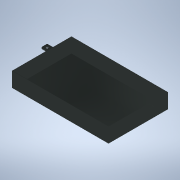
# Autodesk Inventor part: Soporte_Batería
Saved by Autodesk Inventor 2022.1 (Build 261234000, 234)
## iProperties
Part Number: Soporte_Batería
Material: Genérico
Document SubType Name: Modelado
Designer: seb_0
Appearance: Gris plomo - Pulido
Author: seb_0
Autodesk Inventor part; units mm, degrees
ref_plane "Plano YZ" through (0, 0, 0) normal (1, 0, 0) x (0, 1, 0)
ref_plane "Plano XZ" through (0, 0, 0) normal (0, 1, 0) x (-1, 0, 0)
ref_plane "Plano XY" through (0, 0, 0) normal (0, 0, 1) x (1, 0, 0)
sketch "Boceto1" plane through (0, 0, 0) normal (0, 1, 0) x (-1, 0, 0)
  line L0 (0, 0) -> (330.2, 0)
  line L1 (330.2, 0) -> (330.2, -200.66)
  line L2 (330.2, -200.66) -> (0, -200.66)
  line L3 (0, -200.66) -> (0, 0)
  line L4 (-1, -201.66) -> (331.2, -201.66)
  line L5 (331.2, -201.66) -> (331.2, 1)
  line L6 (331.2, 1) -> (-1, 1)
  line L7 (-1, 1) -> (-1, -201.66)
  dimension "d0" = 200.66
  dimension "d1" = 330.2
  dimension "d2" = 1
  constraints: 16 end point, 4 parallel, 2 perpendicular, 1 horizontal, 3 other
  measures "d0" distance of L2.end L0.start
  measures "d1" distance of L1.end L2.end
  measures "d2" distance between parallel lines of L2 L4
extrude "Extrusión1" add sketch "Boceto1" along normal blind 50
sketch "Boceto2" plane through (0, 0, 0) normal (0, -1, 0) x (1, 0, 0)
  line L0 (-331.2, 1) -> (1, 1) projected
  line L1 (1, 1) -> (1, -201.66) projected
  line L2 (-331.2, -201.66) -> (-331.2, 1) projected
  line L3 (1, -201.66) -> (-331.2, -201.66) projected
  point P0 (0, 0)
extrude "Extrusión2" add sketch "Boceto2" along normal blind 1
sketch "Boceto3" plane through (0, 50, 0) normal (0, 1, 0) x (1, 0, 0)
  line L0 (1, -1) -> (1, 201.66) projected
  line L1 (1, 140) -> (21, 140)
  line L2 (21, 140) -> (21, 120)
  line L3 (21, 120) -> (1, 120)
  line L4 (1, 120) -> (1, 140)
  line L5 (-331.2, -1) -> (1, -1) projected
  line L6 (-331.2, 201.66) -> (-331.2, -1) projected
  line L7 (-331.2, 140) -> (-351.2, 140)
  line L8 (-351.2, 140) -> (-351.2, 120)
  line L9 (-351.2, 120) -> (-331.2, 120)
  line L10 (-331.2, 120) -> (-331.2, 140)
  circle A0 centre (11, 130) radius 5
  line L11 (1, 140) -> (21, 120)
  line L12 (21, 140) -> (1, 120)
  line L13 (-351.2, 140) -> (-331.2, 120)
  line L14 (-331.2, 140) -> (-351.2, 120)
  circle A1 centre (-341.2, 130) radius 5
  point P0 (0, 0)
  point P1 (1, 120)
  dimension "d7" = 20
  dimension "d8" = 20
  dimension "d9" = 121
  dimension "d10" = 20
  dimension "d11" = 20
  dimension "d12" = 121
  dimension "d15" = 10
  dimension "d16" = 10
  constraints: 24 end point, 4 parallel, 3 perpendicular, 3 point on line, 2 centre point, 2 horizontal, 2 midpoint, 1 coincident
  measures "d7" distance of L2.end L3.end
  measures "d8" distance of L1.end L2.end
  measures "d9" distance between parallel lines of L5 L3
  measures "d10" distance of L7.start L7.end
  measures "d11" distance of L7.end L8.end
  measures "d12" distance between parallel lines of L5 L9
  measures "d15" diameter of A0
  measures "d16" diameter of A1
extrude "Extrusión3" add sketch "Boceto3" against normal blind 5 contours L12 A0 L11 L3 | L0 L11 A0 L12 | L1 L12 A0 L11 | L11 A0 L12 L2 | L14 A1 L13 L7 | L6 L13 A1 L14 | L9 L14 A1 L13 | L13 A1 L14 L8
fillet "Empalme1" radius 2.5 4 edges at (-351.2, 47.5, -120) (-351.2, 47.5, -140) (21, 47.5, -120) (21, 47.5, -140)
